Autodesk Fusion 360 part; units mm, degrees
note: some values were not read from the file. Chosen so that the rebuilt part matches the saved one: a direction. Set by a fixed rule: which sketch regions a step uses.
(part 4 of 8)
sketch "Sketch6" plane through (0, 6, 0) normal (0, 1, 0) x (-1, 0, 0)
  arc A0 (-5.2505, -46.5856) -> (-4.5189, -45.8544) centre (-13.5, -37.5997) ccw
  arc A1 (-4.3782, -45.8479) -> (-4.5189, -45.8544) centre (-4.4452, -45.922) ccw
  line L0 (-4.3782, -45.8479) -> (-4.0905, -46.108)
  spline S0 degree 5 poles (-4.0905, -46.108) (-4.0863, -46.1118) (-4.0778, -46.1193) (-4.0648, -46.1302) (-4.047, -46.1441) (-4.024, -46.1606) (-4.0005, -46.1765) (-3.9766, -46.192) (-3.9526, -46.2074) (-3.9285, -46.2225) (-3.9042, -46.2376) (-3.8798, -46.2524) (-3.8552, -46.267) (-3.8303, -46.2814) (-3.8052, -46.2954) (-3.7799, -46.3091) (-3.7544, -46.3225) (-3.7287, -46.3358) (-3.7029, -46.3489) (-3.677, -46.3618) (-3.6509, -46.3746) (-3.6247, -46.3871) (-3.5984, -46.3995) (-3.5719, -46.4117) (-3.5453, -46.4237) (-3.5185, -46.4355) (-3.4916, -46.4471) (-3.4646, -46.4586) (-3.4374, -46.4699) (-3.4102, -46.4811) (-3.3828, -46.492) (-3.3554, -46.5029) (-3.3278, -46.5135) (-3.3001, -46.524) (-3.2723, -46.5344) (-3.2443, -46.5445) (-3.2163, -46.5546) (-3.1882, -46.5645) (-3.16, -46.5742) (-3.1316, -46.5838) (-3.1032, -46.5932) (-3.0747, -46.6025) (-3.0461, -46.6116) (-3.0174, -46.6206) (-2.9886, -46.6295) (-2.9597, -46.6382) (-2.9307, -46.6468) (-2.9017, -46.6552) (-2.8725, -46.6635) (-2.8433, -46.6716) (-2.8139, -46.6796) (-2.7845, -46.6875) (-2.755, -46.6953) (-2.7255, -46.7029) (-2.6958, -46.7103) (-2.6661, -46.7176) (-2.6363, -46.7248) (-2.6064, -46.7319) (-2.5764, -46.7388) (-2.5464, -46.7456) (-2.5163, -46.7523) (-2.4861, -46.7588) (-2.4558, -46.7652) (-2.4255, -46.7715) (-2.395, -46.7776) (-2.3646, -46.7836) (-2.334, -46.7895) (-2.3034, -46.7953) (-2.2727, -46.8009) (-2.242, -46.8064) (-2.2111, -46.8117) (-2.1864, -46.8159) (-2.1679, -46.819) (-2.1555, -46.821) (-2.1493, -46.8221) knots 0 0 0 0 0 0 0.01428571 0.02857143 0.04285714 0.05714286 0.07142857 0.08571429 0.1 0.11428571 0.12857143 0.14285714 0.15714286 0.17142857 0.18571429 0.2 0.21428571 0.22857143 0.24285714 0.25714286 0.27142857 0.28571429 0.3 0.31428571 0.32857143 0.34285714 0.35714286 0.37142857 0.38571429 0.4 0.41428571 0.42857143 0.44285714 0.45714286 0.47142857 0.48571429 0.5 0.51428571 0.52857143 0.54285714 0.55714286 0.57142857 0.58571429 0.6 0.61428571 0.62857143 0.64285714 0.65714286 0.67142857 0.68571429 0.7 0.71428571 0.72857143 0.74285714 0.75714286 0.77142857 0.78571429 0.8 0.81428571 0.82857143 0.84285714 0.85714286 0.87142857 0.88571429 0.9 0.91428571 0.92857143 0.94285714 0.95714286 0.97142857 0.98571429 1 1 1 1 1 1
  arc A2 (-2.1493, -46.8221) -> (-1.6591, -46.1836) centre (-13.5, -37.5997) ccw
  spline S1 degree 5 poles (-1.6591, -46.1836) (-1.6617, -46.1779) (-1.6668, -46.1665) (-1.6746, -46.1493) (-1.685, -46.1265) (-1.6982, -46.0981) (-1.7114, -46.0698) (-1.7248, -46.0416) (-1.7383, -46.0136) (-1.7518, -45.9856) (-1.7655, -45.9577) (-1.7793, -45.9299) (-1.7932, -45.9022) (-1.8072, -45.8746) (-1.8213, -45.8471) (-1.8355, -45.8197) (-1.8498, -45.7925) (-1.8642, -45.7653) (-1.8788, -45.7383) (-1.8934, -45.7113) (-1.9082, -45.6845) (-1.9231, -45.6578) (-1.938, -45.6312) (-1.9531, -45.6047) (-1.9683, -45.5783) (-1.9836, -45.552) (-1.9991, -45.5259) (-2.0146, -45.4999) (-2.0302, -45.474) (-2.046, -45.4482) (-2.0619, -45.4225) (-2.0779, -45.397) (-2.094, -45.3716) (-2.1102, -45.3463) (-2.1265, -45.3211) (-2.143, -45.2961) (-2.1596, -45.2712) (-2.1763, -45.2465) (-2.1931, -45.2219) (-2.21, -45.1974) (-2.227, -45.173) (-2.2442, -45.1488) (-2.2615, -45.1248) (-2.2789, -45.1009) (-2.2965, -45.0771) (-2.3142, -45.0535) (-2.332, -45.0301) (-2.3499, -45.0068) (-2.368, -44.9837) (-2.3861, -44.9607) (-2.4045, -44.9379) (-2.4229, -44.9152) (-2.4415, -44.8928) (-2.4603, -44.8705) (-2.4792, -44.8485) (-2.4983, -44.8266) (-2.5175, -44.8049) (-2.5368, -44.7833) (-2.5562, -44.7619) (-2.5758, -44.7408) (-2.5956, -44.7199) (-2.6156, -44.6992) (-2.6358, -44.6789) (-2.6563, -44.6589) (-2.677, -44.6392) (-2.6978, -44.6196) (-2.7187, -44.6002) (-2.7397, -44.581) (-2.7608, -44.562) (-2.7822, -44.5434) (-2.8041, -44.5254) (-2.8222, -44.5118) (-2.8361, -44.502) (-2.8455, -44.4958) (-2.8502, -44.4927) knots -1 -1 -1 -1 -1 -1 -0.98571429 -0.97142857 -0.95714286 -0.94285714 -0.92857143 -0.91428571 -0.9 -0.88571429 -0.87142857 -0.85714286 -0.84285714 -0.82857143 -0.81428571 -0.8 -0.78571429 -0.77142857 -0.75714286 -0.74285714 -0.72857143 -0.71428571 -0.7 -0.68571429 -0.67142857 -0.65714286 -0.64285714 -0.62857143 -0.61428571 -0.6 -0.58571429 -0.57142857 -0.55714286 -0.54285714 -0.52857143 -0.51428571 -0.5 -0.48571429 -0.47142857 -0.45714286 -0.44285714 -0.42857143 -0.41428571 -0.4 -0.38571429 -0.37142857 -0.35714286 -0.34285714 -0.32857143 -0.31428571 -0.3 -0.28571429 -0.27142857 -0.25714286 -0.24285714 -0.22857143 -0.21428571 -0.2 -0.18571429 -0.17142857 -0.15714286 -0.14285714 -0.12857143 -0.11428571 -0.1 -0.08571429 -0.07142857 -0.05714286 -0.04285714 -0.02857143 -0.01428571 0 0 0 0 0 0
  line L1 (-2.8502, -44.4927) -> (-3.1759, -44.2819)
  arc A3 (-3.2059, -44.1443) -> (-3.1759, -44.2819) centre (-3.1215, -44.198) ccw
  arc A4 (-3.2059, -44.1443) -> (-2.6884, -43.2486) centre (-13.5, -37.5997) ccw
  arc A5 (-2.5542, -43.2059) -> (-2.6884, -43.2486) centre (-2.5998, -43.2949) ccw
  line L2 (-2.5542, -43.2059) -> (-2.209, -43.3827)
  spline S2 degree 5 poles (-2.209, -43.3827) (-2.2039, -43.3853) (-2.1938, -43.3904) (-2.1784, -43.3975) (-2.1576, -43.4063) (-2.1311, -43.4163) (-2.1043, -43.4256) (-2.0773, -43.4344) (-2.0501, -43.443) (-2.0229, -43.4514) (-1.9955, -43.4597) (-1.9681, -43.4677) (-1.9406, -43.4755) (-1.9129, -43.4828) (-1.885, -43.4899) (-1.857, -43.4966) (-1.8289, -43.503) (-1.8006, -43.5091) (-1.7723, -43.5151) (-1.7439, -43.5209) (-1.7154, -43.5264) (-1.6869, -43.5318) (-1.6582, -43.5369) (-1.6295, -43.5419) (-1.6007, -43.5466) (-1.5717, -43.551) (-1.5427, -43.5553) (-1.5137, -43.5594) (-1.4845, -43.5633) (-1.4553, -43.567) (-1.4261, -43.5705) (-1.3967, -43.5739) (-1.3673, -43.577) (-1.3378, -43.58) (-1.3083, -43.5828) (-1.2787, -43.5854) (-1.249, -43.5878) (-1.2193, -43.5901) (-1.1895, -43.5922) (-1.1597, -43.5941) (-1.1298, -43.5959) (-1.0998, -43.5975) (-1.0698, -43.5989) (-1.0398, -43.6002) (-1.0097, -43.6013) (-0.9795, -43.6022) (-0.9493, -43.603) (-0.9191, -43.6036) (-0.8888, -43.604) (-0.8584, -43.6043) (-0.828, -43.6045) (-0.7976, -43.6045) (-0.7671, -43.6043) (-0.7365, -43.604) (-0.706, -43.6036) (-0.6753, -43.6029) (-0.6447, -43.6022) (-0.614, -43.6012) (-0.5833, -43.6002) (-0.5525, -43.599) (-0.5217, -43.5976) (-0.4908, -43.5961) (-0.4599, -43.5945) (-0.429, -43.5927) (-0.398, -43.5907) (-0.367, -43.5886) (-0.336, -43.5864) (-0.3049, -43.584) (-0.2738, -43.5815) (-0.2427, -43.5789) (-0.2115, -43.5761) (-0.1866, -43.5737) (-0.1679, -43.5719) (-0.1554, -43.5707) (-0.1491, -43.57) knots 0 0 0 0 0 0 0.01428571 0.02857143 0.04285714 0.05714286 0.07142857 0.08571429 0.1 0.11428571 0.12857143 0.14285714 0.15714286 0.17142857 0.18571429 0.2 0.21428571 0.22857143 0.24285714 0.25714286 0.27142857 0.28571429 0.3 0.31428571 0.32857143 0.34285714 0.35714286 0.37142857 0.38571429 0.4 0.41428571 0.42857143 0.44285714 0.45714286 0.47142857 0.48571429 0.5 0.51428571 0.52857143 0.54285714 0.55714286 0.57142857 0.58571429 0.6 0.61428571 0.62857143 0.64285714 0.65714286 0.67142857 0.68571429 0.7 0.71428571 0.72857143 0.74285714 0.75714286 0.77142857 0.78571429 0.8 0.81428571 0.82857143 0.84285714 0.85714286 0.87142857 0.88571429 0.9 0.91428571 0.92857143 0.94285714 0.95714286 0.97142857 0.98571429 1 1 1 1 1 1
  arc A6 (-0.1491, -43.57) -> (0.1591, -42.8265) centre (-13.5, -37.5997) ccw
  spline S3 degree 5 poles (0.1591, -42.8265) (0.1551, -42.8216) (0.1472, -42.8119) (0.1353, -42.7974) (0.1193, -42.778) (0.0992, -42.754) (0.0791, -42.7301) (0.0589, -42.7063) (0.0386, -42.6827) (0.0183, -42.6592) (-0.0021, -42.6358) (-0.0227, -42.6125) (-0.0432, -42.5893) (-0.0639, -42.5663) (-0.0846, -42.5434) (-0.1055, -42.5206) (-0.1263, -42.498) (-0.1473, -42.4755) (-0.1684, -42.4531) (-0.1895, -42.4309) (-0.2107, -42.4088) (-0.232, -42.3869) (-0.2533, -42.365) (-0.2747, -42.3433) (-0.2963, -42.3218) (-0.3178, -42.3004) (-0.3395, -42.2791) (-0.3612, -42.258) (-0.3831, -42.2371) (-0.405, -42.2162) (-0.4269, -42.1956) (-0.449, -42.175) (-0.4711, -42.1547) (-0.4933, -42.1344) (-0.5156, -42.1144) (-0.538, -42.0945) (-0.5605, -42.0747) (-0.583, -42.0551) (-0.6056, -42.0357) (-0.6283, -42.0164) (-0.651, -41.9973) (-0.6739, -41.9784) (-0.6968, -41.9597) (-0.7198, -41.9411) (-0.7429, -41.9227) (-0.7661, -41.9045) (-0.7894, -41.8864) (-0.8127, -41.8685) (-0.8362, -41.8509) (-0.8597, -41.8334) (-0.8833, -41.8161) (-0.907, -41.799) (-0.9308, -41.7822) (-0.9547, -41.7655) (-0.9786, -41.7491) (-1.0027, -41.7329) (-1.0268, -41.7169) (-1.0511, -41.701) (-1.0754, -41.6854) (-1.0998, -41.6701) (-1.1243, -41.655) (-1.149, -41.6402) (-1.1738, -41.6258) (-1.1987, -41.6118) (-1.2238, -41.5981) (-1.249, -41.5846) (-1.2742, -41.5713) (-1.2994, -41.5581) (-1.3248, -41.5452) (-1.3503, -41.5328) (-1.3761, -41.5211) (-1.397, -41.5126) (-1.413, -41.5068) (-1.4237, -41.5032) (-1.4291, -41.5015) knots -1 -1 -1 -1 -1 -1 -0.98571429 -0.97142857 -0.95714286 -0.94285714 -0.92857143 -0.91428571 -0.9 -0.88571429 -0.87142857 -0.85714286 -0.84285714 -0.82857143 -0.81428571 -0.8 -0.78571429 -0.77142857 -0.75714286 -0.74285714 -0.72857143 -0.71428571 -0.7 -0.68571429 -0.67142857 -0.65714286 -0.64285714 -0.62857143 -0.61428571 -0.6 -0.58571429 -0.57142857 -0.55714286 -0.54285714 -0.52857143 -0.51428571 -0.5 -0.48571429 -0.47142857 -0.45714286 -0.44285714 -0.42857143 -0.41428571 -0.4 -0.38571429 -0.37142857 -0.35714286 -0.34285714 -0.32857143 -0.31428571 -0.3 -0.28571429 -0.27142857 -0.25714286 -0.24285714 -0.22857143 -0.21428571 -0.2 -0.18571429 -0.17142857 -0.15714286 -0.14285714 -0.12857143 -0.11428571 -0.1 -0.08571429 -0.07142857 -0.05714286 -0.04285714 -0.02857143 -0.01428571 0 0 0 0 0 0
  line L3 (-1.4291, -41.5015) -> (-1.7982, -41.3822)
  arc A7 (-1.8628, -41.257) -> (-1.7982, -41.3822) centre (-1.7674, -41.287) ccw
  arc A8 (-1.8628, -41.257) -> (-1.5948, -40.2579) centre (-13.5, -37.5997) ccw
  arc A9 (-1.4762, -40.1819) -> (-1.5948, -40.2579) centre (-1.4972, -40.2797) ccw
  line L4 (-1.4762, -40.1819) -> (-1.0969, -40.2634)
  spline S4 degree 5 poles (-1.0969, -40.2634) (-1.0914, -40.2645) (-1.0803, -40.2668) (-1.0636, -40.2697) (-1.0412, -40.2728) (-1.0131, -40.2757) (-0.9847, -40.2777) (-0.9563, -40.2792) (-0.9279, -40.2805) (-0.8994, -40.2815) (-0.8709, -40.2824) (-0.8423, -40.2831) (-0.8137, -40.2834) (-0.785, -40.2834) (-0.7563, -40.283) (-0.7275, -40.2822) (-0.6987, -40.2811) (-0.6698, -40.2798) (-0.6409, -40.2782) (-0.612, -40.2764) (-0.583, -40.2744) (-0.5541, -40.2722) (-0.5251, -40.2698) (-0.496, -40.2671) (-0.467, -40.2641) (-0.4379, -40.261) (-0.4088, -40.2576) (-0.3796, -40.254) (-0.3505, -40.2503) (-0.3213, -40.2463) (-0.2921, -40.2421) (-0.2629, -40.2377) (-0.2337, -40.2332) (-0.2044, -40.2284) (-0.1752, -40.2235) (-0.1459, -40.2183) (-0.1166, -40.213) (-0.0873, -40.2075) (-0.058, -40.2018) (-0.0287, -40.196) (0.0006, -40.1899) (0.03, -40.1837) (0.0593, -40.1773) (0.0887, -40.1708) (0.118, -40.164) (0.1474, -40.1571) (0.1768, -40.1501) (0.2062, -40.1428) (0.2356, -40.1354) (0.265, -40.1279) (0.2944, -40.1201) (0.3238, -40.1122) (0.3532, -40.1042) (0.3826, -40.096) (0.412, -40.0876) (0.4414, -40.0791) (0.4708, -40.0704) (0.5002, -40.0616) (0.5297, -40.0526) (0.5591, -40.0435) (0.5885, -40.0342) (0.6179, -40.0248) (0.6473, -40.0152) (0.6767, -40.0054) (0.7061, -39.9955) (0.7355, -39.9855) (0.7649, -39.9753) (0.7943, -39.965) (0.8237, -39.9545) (0.8531, -39.9439) (0.8825, -39.9331) (0.906, -39.9244) (0.9236, -39.9178) (0.9353, -39.9134) (0.9412, -39.9111) knots 0 0 0 0 0 0 0.01428571 0.02857143 0.04285714 0.05714286 0.07142857 0.08571429 0.1 0.11428571 0.12857143 0.14285714 0.15714286 0.17142857 0.18571429 0.2 0.21428571 0.22857143 0.24285714 0.25714286 0.27142857 0.28571429 0.3 0.31428571 0.32857143 0.34285714 0.35714286 0.37142857 0.38571429 0.4 0.41428571 0.42857143 0.44285714 0.45714286 0.47142857 0.48571429 0.5 0.51428571 0.52857143 0.54285714 0.55714286 0.57142857 0.58571429 0.6 0.61428571 0.62857143 0.64285714 0.65714286 0.67142857 0.68571429 0.7 0.71428571 0.72857143 0.74285714 0.75714286 0.77142857 0.78571429 0.8 0.81428571 0.82857143 0.84285714 0.85714286 0.87142857 0.88571429 0.9 0.91428571 0.92857143 0.94285714 0.95714286 0.97142857 0.98571429 1 1 1 1 1 1
  arc A10 (0.9412, -39.9111) -> (1.0465, -39.1132) centre (-13.5, -37.5997) ccw
  spline S5 degree 5 poles (1.0465, -39.1132) (1.0414, -39.1095) (1.0312, -39.1021) (1.0159, -39.0912) (0.9955, -39.0767) (0.9699, -39.0587) (0.9443, -39.0408) (0.9186, -39.023) (0.8929, -39.0054) (0.8671, -38.988) (0.8413, -38.9707) (0.8155, -38.9535) (0.7896, -38.9364) (0.7637, -38.9196) (0.7378, -38.9028) (0.7118, -38.8862) (0.6857, -38.8698) (0.6597, -38.8534) (0.6335, -38.8373) (0.6074, -38.8213) (0.5812, -38.8054) (0.5549, -38.7897) (0.5287, -38.7742) (0.5024, -38.7588) (0.476, -38.7435) (0.4496, -38.7284) (0.4232, -38.7135) (0.3967, -38.6987) (0.3702, -38.6841) (0.3437, -38.6697) (0.3171, -38.6554) (0.2905, -38.6413) (0.2638, -38.6273) (0.2371, -38.6135) (0.2104, -38.5999) (0.1837, -38.5865) (0.1569, -38.5732) (0.13, -38.5601) (0.1032, -38.5472) (0.0763, -38.5345) (0.0493, -38.5219) (0.0224, -38.5096) (-0.0047, -38.4974) (-0.0317, -38.4854) (-0.0588, -38.4736) (-0.0859, -38.462) (-0.113, -38.4506) (-0.1402, -38.4394) (-0.1674, -38.4284) (-0.1946, -38.4176) (-0.2219, -38.407) (-0.2492, -38.3966) (-0.2766, -38.3865) (-0.3039, -38.3766) (-0.3313, -38.3669) (-0.3588, -38.3575) (-0.3863, -38.3483) (-0.4138, -38.3393) (-0.4413, -38.3305) (-0.4688, -38.322) (-0.4964, -38.3137) (-0.5241, -38.3059) (-0.5518, -38.2984) (-0.5795, -38.2913) (-0.6073, -38.2845) (-0.635, -38.278) (-0.6628, -38.2717) (-0.6906, -38.2655) (-0.7185, -38.2596) (-0.7463, -38.2542) (-0.7743, -38.2496) (-0.7967, -38.2468) (-0.8136, -38.2453) (-0.8249, -38.2446) (-0.8305, -38.2443) knots -1 -1 -1 -1 -1 -1 -0.98571429 -0.97142857 -0.95714286 -0.94285714 -0.92857143 -0.91428571 -0.9 -0.88571429 -0.87142857 -0.85714286 -0.84285714 -0.82857143 -0.81428571 -0.8 -0.78571429 -0.77142857 -0.75714286 -0.74285714 -0.72857143 -0.71428571 -0.7 -0.68571429 -0.67142857 -0.65714286 -0.64285714 -0.62857143 -0.61428571 -0.6 -0.58571429 -0.57142857 -0.55714286 -0.54285714 -0.52857143 -0.51428571 -0.5 -0.48571429 -0.47142857 -0.45714286 -0.44285714 -0.42857143 -0.41428571 -0.4 -0.38571429 -0.37142857 -0.35714286 -0.34285714 -0.32857143 -0.31428571 -0.3 -0.28571429 -0.27142857 -0.25714286 -0.24285714 -0.22857143 -0.21428571 -0.2 -0.18571429 -0.17142857 -0.15714286 -0.14285714 -0.12857143 -0.11428571 -0.1 -0.08571429 -0.07142857 -0.05714286 -0.04285714 -0.02857143 -0.01428571 0 0 0 0 0 0
  line L5 (-0.8305, -38.2443) -> (-1.2179, -38.2246)
  arc A11 (-1.3127, -38.1205) -> (-1.2179, -38.2246) centre (-1.2128, -38.1247) ccw
  arc A12 (-1.3127, -38.1205) -> (-1.3124, -37.086) centre (-13.5, -37.5997) ccw
  arc A13 (-1.2176, -36.9819) -> (-1.3124, -37.086) centre (-1.2125, -37.0818) ccw
  line L6 (-1.2176, -36.9819) -> (-0.8302, -36.9624)
  spline S6 degree 5 poles (-0.8302, -36.9624) (-0.8245, -36.9622) (-0.8132, -36.9615) (-0.7963, -36.96) (-0.7739, -36.9572) (-0.746, -36.9526) (-0.7181, -36.9472) (-0.6903, -36.9414) (-0.6625, -36.9352) (-0.6347, -36.9289) (-0.6069, -36.9224) (-0.5791, -36.9156) (-0.5514, -36.9085) (-0.5237, -36.9011) (-0.496, -36.8932) (-0.4684, -36.885) (-0.4409, -36.8765) (-0.4133, -36.8677) (-0.3858, -36.8587) (-0.3584, -36.8495) (-0.3309, -36.8401) (-0.3035, -36.8305) (-0.2761, -36.8206) (-0.2488, -36.8105) (-0.2214, -36.8002) (-0.1942, -36.7896) (-0.1669, -36.7788) (-0.1397, -36.7678) (-0.1125, -36.7566) (-0.0854, -36.7452) (-0.0583, -36.7336) (-0.0312, -36.7218) (-0.0041, -36.7099) (0.0229, -36.6977) (0.0499, -36.6854) (0.0768, -36.6728) (0.1037, -36.6601) (0.1306, -36.6472) (0.1574, -36.6341) (0.1842, -36.6209) (0.211, -36.6074) (0.2377, -36.5938) (0.2644, -36.5801) (0.2911, -36.5661) (0.3177, -36.552) (0.3443, -36.5378) (0.3708, -36.5233) (0.3974, -36.5087) (0.4238, -36.494) (0.4503, -36.4791) (0.4767, -36.464) (0.503, -36.4488) (0.5293, -36.4334) (0.5556, -36.4179) (0.5819, -36.4022) (0.6081, -36.3863) (0.6343, -36.3703) (0.6604, -36.3542) (0.6865, -36.3379) (0.7125, -36.3215) (0.7385, -36.3049) (0.7645, -36.2881) (0.7904, -36.2713) (0.8163, -36.2542) (0.8421, -36.2371) (0.8679, -36.2198) (0.8937, -36.2023) (0.9194, -36.1847) (0.9451, -36.167) (0.9707, -36.1492) (0.9963, -36.1312) (1.0168, -36.1166) (1.0321, -36.1057) (1.0423, -36.0984) (1.0474, -36.0947) knots 0 0 0 0 0 0 0.01428571 0.02857143 0.04285714 0.05714286 0.07142857 0.08571429 0.1 0.11428571 0.12857143 0.14285714 0.15714286 0.17142857 0.18571429 0.2 0.21428571 0.22857143 0.24285714 0.25714286 0.27142857 0.28571429 0.3 0.31428571 0.32857143 0.34285714 0.35714286 0.37142857 0.38571429 0.4 0.41428571 0.42857143 0.44285714 0.45714286 0.47142857 0.48571429 0.5 0.51428571 0.52857143 0.54285714 0.55714286 0.57142857 0.58571429 0.6 0.61428571 0.62857143 0.64285714 0.65714286 0.67142857 0.68571429 0.7 0.71428571 0.72857143 0.74285714 0.75714286 0.77142857 0.78571429 0.8 0.81428571 0.82857143 0.84285714 0.85714286 0.87142857 0.88571429 0.9 0.91428571 0.92857143 0.94285714 0.95714286 0.97142857 0.98571429 1 1 1 1 1 1
  arc A14 (1.0474, -36.0947) -> (0.9425, -35.2967) centre (-13.5, -37.5997) ccw
  spline S7 degree 5 poles (0.9425, -35.2967) (0.9367, -35.2944) (0.9249, -35.29) (0.9073, -35.2834) (0.8838, -35.2746) (0.8544, -35.2639) (0.8251, -35.2532) (0.7957, -35.2427) (0.7663, -35.2324) (0.7369, -35.2222) (0.7075, -35.2121) (0.6781, -35.2022) (0.6487, -35.1925) (0.6193, -35.1829) (0.5899, -35.1734) (0.5605, -35.1641) (0.5311, -35.1549) (0.5017, -35.1459) (0.4723, -35.1371) (0.4428, -35.1284) (0.4134, -35.1199) (0.384, -35.1115) (0.3546, -35.1033) (0.3252, -35.0952) (0.2958, -35.0873) (0.2664, -35.0795) (0.237, -35.072) (0.2076, -35.0646) (0.1783, -35.0573) (0.1489, -35.0502) (0.1195, -35.0433) (0.0902, -35.0366) (0.0608, -35.03) (0.0315, -35.0236) (0.0021, -35.0173) (-0.0272, -35.0113) (-0.0565, -35.0054) (-0.0858, -34.9997) (-0.1151, -34.9942) (-0.1444, -34.9888) (-0.1737, -34.9837) (-0.2029, -34.9787) (-0.2322, -34.9739) (-0.2614, -34.9694) (-0.2906, -34.965) (-0.3198, -34.9608) (-0.3489, -34.9568) (-0.3781, -34.953) (-0.4072, -34.9494) (-0.4363, -34.946) (-0.4654, -34.9428) (-0.4945, -34.9399) (-0.5235, -34.9372) (-0.5525, -34.9347) (-0.5815, -34.9325) (-0.6104, -34.9305) (-0.6394, -34.9287) (-0.6682, -34.9271) (-0.6971, -34.9257) (-0.7259, -34.9246) (-0.7547, -34.9238) (-0.7835, -34.9234) (-0.8121, -34.9233) (-0.8408, -34.9237) (-0.8693, -34.9243) (-0.8979, -34.9252) (-0.9263, -34.9263) (-0.9548, -34.9275) (-0.9832, -34.929) (-1.0115, -34.931) (-1.0397, -34.9338) (-1.0621, -34.9369) (-1.0788, -34.9398) (-1.0899, -34.9421) (-1.0954, -34.9433) knots -1 -1 -1 -1 -1 -1 -0.98571429 -0.97142857 -0.95714286 -0.94285714 -0.92857143 -0.91428571 -0.9 -0.88571429 -0.87142857 -0.85714286 -0.84285714 -0.82857143 -0.81428571 -0.8 -0.78571429 -0.77142857 -0.75714286 -0.74285714 -0.72857143 -0.71428571 -0.7 -0.68571429 -0.67142857 -0.65714286 -0.64285714 -0.62857143 -0.61428571 -0.6 -0.58571429 -0.57142857 -0.55714286 -0.54285714 -0.52857143 -0.51428571 -0.5 -0.48571429 -0.47142857 -0.45714286 -0.44285714 -0.42857143 -0.41428571 -0.4 -0.38571429 -0.37142857 -0.35714286 -0.34285714 -0.32857143 -0.31428571 -0.3 -0.28571429 -0.27142857 -0.25714286 -0.24285714 -0.22857143 -0.21428571 -0.2 -0.18571429 -0.17142857 -0.15714286 -0.14285714 -0.12857143 -0.11428571 -0.1 -0.08571429 -0.07142857 -0.05714286 -0.04285714 -0.02857143 -0.01428571 0 0 0 0 0 0
  line L7 (-1.0954, -34.9433) -> (-1.4747, -35.0245)
  arc A15 (-1.5932, -34.9484) -> (-1.4747, -35.0245) centre (-1.4956, -34.9267) ccw
  arc A16 (-1.5932, -34.9484) -> (-1.8607, -33.9492) centre (-13.5, -37.5997) ccw
  arc A17 (-1.796, -33.8241) -> (-1.8607, -33.9492) centre (-1.7653, -33.9192) ccw
  line L8 (-1.796, -33.8241) -> (-1.4268, -33.705)
  spline S8 degree 5 poles (-1.4268, -33.705) (-1.4214, -33.7032) (-1.4107, -33.6996) (-1.3948, -33.6938) (-1.3738, -33.6853) (-1.348, -33.6737) (-1.3225, -33.6613) (-1.2971, -33.6484) (-1.2719, -33.6353) (-1.2466, -33.6219) (-1.2215, -33.6085) (-1.1964, -33.5948) (-1.1715, -33.5807) (-1.1467, -33.5664) (-1.122, -33.5516) (-1.0974, -33.5366) (-1.073, -33.5212) (-1.0487, -33.5056) (-1.0245, -33.4898) (-1.0003, -33.4738) (-0.9762, -33.4576) (-0.9522, -33.4412) (-0.9283, -33.4246) (-0.9045, -33.4077) (-0.8808, -33.3907) (-0.8572, -33.3734) (-0.8337, -33.3559) (-0.8103, -33.3382) (-0.7869, -33.3204) (-0.7636, -33.3024) (-0.7404, -33.2841) (-0.7173, -33.2658) (-0.6943, -33.2472) (-0.6714, -33.2285) (-0.6485, -33.2095) (-0.6257, -33.1905) (-0.603, -33.1712) (-0.5804, -33.1518) (-0.5579, -33.1322) (-0.5354, -33.1125) (-0.513, -33.0926) (-0.4907, -33.0725) (-0.4685, -33.0523) (-0.4463, -33.032) (-0.4243, -33.0115) (-0.4023, -32.9908) (-0.3804, -32.97) (-0.3586, -32.949) (-0.3368, -32.9279) (-0.3151, -32.9067) (-0.2935, -32.8853) (-0.272, -32.8637) (-0.2506, -32.8421) (-0.2292, -32.8203) (-0.2079, -32.7983) (-0.1867, -32.7762) (-0.1655, -32.754) (-0.1445, -32.7317) (-0.1235, -32.7092) (-0.1026, -32.6865) (-0.0818, -32.6638) (-0.061, -32.6409) (-0.0403, -32.6179) (-0.0198, -32.5948) (0.0008, -32.5715) (0.0212, -32.5481) (0.0416, -32.5246) (0.0619, -32.5009) (0.0821, -32.4772) (0.1022, -32.4533) (0.1223, -32.4293) (0.1383, -32.41) (0.1502, -32.3954) (0.1582, -32.3857) (0.1621, -32.3809) knots 0 0 0 0 0 0 0.01428571 0.02857143 0.04285714 0.05714286 0.07142857 0.08571429 0.1 0.11428571 0.12857143 0.14285714 0.15714286 0.17142857 0.18571429 0.2 0.21428571 0.22857143 0.24285714 0.25714286 0.27142857 0.28571429 0.3 0.31428571 0.32857143 0.34285714 0.35714286 0.37142857 0.38571429 0.4 0.41428571 0.42857143 0.44285714 0.45714286 0.47142857 0.48571429 0.5 0.51428571 0.52857143 0.54285714 0.55714286 0.57142857 0.58571429 0.6 0.61428571 0.62857143 0.64285714 0.65714286 0.67142857 0.68571429 0.7 0.71428571 0.72857143 0.74285714 0.75714286 0.77142857 0.78571429 0.8 0.81428571 0.82857143 0.84285714 0.85714286 0.87142857 0.88571429 0.9 0.91428571 0.92857143 0.94285714 0.95714286 0.97142857 0.98571429 1 1 1 1 1 1
  arc A18 (0.1621, -32.3809) -> (-0.1457, -31.6371) centre (-13.5, -37.5997) ccw
  spline S9 degree 5 poles (-0.1457, -31.6371) (-0.1519, -31.6365) (-0.1644, -31.6353) (-0.1831, -31.6334) (-0.2081, -31.6311) (-0.2392, -31.6283) (-0.2704, -31.6256) (-0.3015, -31.6231) (-0.3325, -31.6207) (-0.3636, -31.6184) (-0.3946, -31.6163) (-0.4255, -31.6144) (-0.4564, -31.6125) (-0.4873, -31.6109) (-0.5182, -31.6093) (-0.549, -31.608) (-0.5798, -31.6067) (-0.6105, -31.6057) (-0.6412, -31.6047) (-0.6719, -31.6039) (-0.7025, -31.6033) (-0.7331, -31.6028) (-0.7636, -31.6025) (-0.7941, -31.6023) (-0.8245, -31.6023) (-0.8549, -31.6024) (-0.8853, -31.6027) (-0.9156, -31.6031) (-0.9458, -31.6037) (-0.976, -31.6045) (-1.0062, -31.6054) (-1.0363, -31.6065) (-1.0664, -31.6077) (-1.0964, -31.6091) (-1.1263, -31.6107) (-1.1562, -31.6125) (-1.1861, -31.6144) (-1.2158, -31.6164) (-1.2456, -31.6187) (-1.2752, -31.6211) (-1.3048, -31.6237) (-1.3344, -31.6265) (-1.3639, -31.6294) (-1.3933, -31.6326) (-1.4226, -31.6359) (-1.4519, -31.6394) (-1.4811, -31.6431) (-1.5102, -31.647) (-1.5393, -31.651) (-1.5683, -31.6553) (-1.5972, -31.6598) (-1.626, -31.6645) (-1.6548, -31.6694) (-1.6834, -31.6745) (-1.712, -31.6798) (-1.7405, -31.6854) (-1.7689, -31.6911) (-1.7972, -31.6971) (-1.8254, -31.7032) (-1.8536, -31.7096) (-1.8816, -31.7163) (-1.9094, -31.7233) (-1.9372, -31.7307) (-1.9647, -31.7384) (-1.9922, -31.7464) (-2.0195, -31.7546) (-2.0467, -31.7631) (-2.0739, -31.7716) (-2.1009, -31.7804) (-2.1278, -31.7897) (-2.1542, -31.7997) (-2.1751, -31.8085) (-2.1904, -31.8156) (-2.2006, -31.8207) (-2.2056, -31.8232) knots -1 -1 -1 -1 -1 -1 -0.98571429 -0.97142857 -0.95714286 -0.94285714 -0.92857143 -0.91428571 -0.9 -0.88571429 -0.87142857 -0.85714286 -0.84285714 -0.82857143 -0.81428571 -0.8 -0.78571429 -0.77142857 -0.75714286 -0.74285714 -0.72857143 -0.71428571 -0.7 -0.68571429 -0.67142857 -0.65714286 -0.64285714 -0.62857143 -0.61428571 -0.6 -0.58571429 -0.57142857 -0.55714286 -0.54285714 -0.52857143 -0.51428571 -0.5 -0.48571429 -0.47142857 -0.45714286 -0.44285714 -0.42857143 -0.41428571 -0.4 -0.38571429 -0.37142857 -0.35714286 -0.34285714 -0.32857143 -0.31428571 -0.3 -0.28571429 -0.27142857 -0.25714286 -0.24285714 -0.22857143 -0.21428571 -0.2 -0.18571429 -0.17142857 -0.15714286 -0.14285714 -0.12857143 -0.11428571 -0.1 -0.08571429 -0.07142857 -0.05714286 -0.04285714 -0.02857143 -0.01428571 0 0 0 0 0 0
  line L9 (-2.2056, -31.8232) -> (-2.551, -31.9999)
  arc A19 (-2.6851, -31.9571) -> (-2.551, -31.9999) centre (-2.5965, -31.9108) ccw
  arc A20 (-2.6851, -31.9571) -> (-3.2021, -31.0611) centre (-13.5, -37.5997) ccw
  arc A21 (-3.172, -30.9235) -> (-3.2021, -31.0611) centre (-3.1177, -31.0075) ccw
  line L10 (-3.172, -30.9235) -> (-2.8462, -30.7129)
  spline S10 degree 5 poles (-2.8462, -30.7129) (-2.8415, -30.7098) (-2.8321, -30.7036) (-2.8182, -30.6938) (-2.8001, -30.6802) (-2.7782, -30.6623) (-2.7568, -30.6437) (-2.7356, -30.6247) (-2.7146, -30.6055) (-2.6937, -30.5861) (-2.6729, -30.5666) (-2.6522, -30.5468) (-2.6317, -30.5268) (-2.6115, -30.5065) (-2.5915, -30.4859) (-2.5717, -30.465) (-2.5521, -30.4438) (-2.5326, -30.4225) (-2.5133, -30.4009) (-2.4941, -30.3792) (-2.475, -30.3573) (-2.4561, -30.3353) (-2.4373, -30.313) (-2.4187, -30.2906) (-2.4002, -30.268) (-2.3819, -30.2452) (-2.3637, -30.2222) (-2.3456, -30.1991) (-2.3277, -30.1758) (-2.3099, -30.1524) (-2.2922, -30.1288) (-2.2746, -30.105) (-2.2572, -30.0812) (-2.2398, -30.0571) (-2.2227, -30.0329) (-2.2056, -30.0086) (-2.1887, -29.9841) (-2.1718, -29.9595) (-2.1551, -29.9348) (-2.1385, -29.9099) (-2.1221, -29.8849) (-2.1057, -29.8597) (-2.0895, -29.8345) (-2.0734, -29.8091) (-2.0574, -29.7836) (-2.0415, -29.7579) (-2.0257, -29.7321) (-2.01, -29.7062) (-1.9945, -29.6802) (-1.979, -29.6541) (-1.9637, -29.6278) (-1.9485, -29.6015) (-1.9334, -29.575) (-1.9184, -29.5484) (-1.9035, -29.5217) (-1.8887, -29.4948) (-1.8741, -29.4679) (-1.8595, -29.4409) (-1.8451, -29.4137) (-1.8307, -29.3865) (-1.8165, -29.3591) (-1.8024, -29.3316) (-1.7884, -29.304) (-1.7745, -29.2764) (-1.7607, -29.2486) (-1.747, -29.2207) (-1.7334, -29.1927) (-1.7199, -29.1646) (-1.7065, -29.1364) (-1.6933, -29.1081) (-1.6801, -29.0798) (-1.6697, -29.057) (-1.6619, -29.0398) (-1.6567, -29.0284) (-1.6541, -29.0227) knots 0 0 0 0 0 0 0.01428571 0.02857143 0.04285714 0.05714286 0.07142857 0.08571429 0.1 0.11428571 0.12857143 0.14285714 0.15714286 0.17142857 0.18571429 0.2 0.21428571 0.22857143 0.24285714 0.25714286 0.27142857 0.28571429 0.3 0.31428571 0.32857143 0.34285714 0.35714286 0.37142857 0.38571429 0.4 0.41428571 0.42857143 0.44285714 0.45714286 0.47142857 0.48571429 0.5 0.51428571 0.52857143 0.54285714 0.55714286 0.57142857 0.58571429 0.6 0.61428571 0.62857143 0.64285714 0.65714286 0.67142857 0.68571429 0.7 0.71428571 0.72857143 0.74285714 0.75714286 0.77142857 0.78571429 0.8 0.81428571 0.82857143 0.84285714 0.85714286 0.87142857 0.88571429 0.9 0.91428571 0.92857143 0.94285714 0.95714286 0.97142857 0.98571429 1 1 1 1 1 1
  arc A22 (-1.6541, -29.0227) -> (-2.1439, -28.384) centre (-13.5, -37.5997) ccw
  spline S11 degree 5 poles (-2.1439, -28.384) (-2.1501, -28.385) (-2.1625, -28.387) (-2.1811, -28.3901) (-2.2058, -28.3942) (-2.2366, -28.3996) (-2.2674, -28.4051) (-2.2981, -28.4107) (-2.3287, -28.4164) (-2.3592, -28.4223) (-2.3897, -28.4283) (-2.4201, -28.4344) (-2.4505, -28.4406) (-2.4808, -28.447) (-2.511, -28.4535) (-2.5411, -28.4602) (-2.5711, -28.4669) (-2.6011, -28.4738) (-2.631, -28.4809) (-2.6608, -28.4881) (-2.6905, -28.4954) (-2.7202, -28.5028) (-2.7498, -28.5104) (-2.7793, -28.5181) (-2.8087, -28.526) (-2.838, -28.534) (-2.8673, -28.5421) (-2.8964, -28.5504) (-2.9255, -28.5588) (-2.9545, -28.5673) (-2.9834, -28.576) (-3.0122, -28.5849) (-3.0409, -28.5939) (-3.0695, -28.603) (-3.098, -28.6123) (-3.1264, -28.6217) (-3.1548, -28.6312) (-3.183, -28.6409) (-3.2111, -28.6508) (-3.2392, -28.6608) (-3.2671, -28.671) (-3.2949, -28.6813) (-3.3226, -28.6918) (-3.3502, -28.7025) (-3.3777, -28.7133) (-3.405, -28.7242) (-3.4323, -28.7354) (-3.4595, -28.7466) (-3.4865, -28.7581) (-3.5134, -28.7697) (-3.5402, -28.7815) (-3.5668, -28.7935) (-3.5933, -28.8057) (-3.6196, -28.818) (-3.6458, -28.8306) (-3.6719, -28.8433) (-3.6979, -28.8562) (-3.7237, -28.8693) (-3.7494, -28.8825) (-3.7749, -28.896) (-3.8002, -28.9097) (-3.8253, -28.9237) (-3.8502, -28.938) (-3.8748, -28.9526) (-3.8992, -28.9674) (-3.9235, -28.9824) (-3.9476, -28.9976) (-3.9716, -29.0129) (-3.9955, -29.0284) (-4.019, -29.0443) (-4.042, -29.0608) (-4.0598, -29.0747) (-4.0728, -29.0856) (-4.0813, -29.0931) (-4.0855, -29.0969) knots -1 -1 -1 -1 -1 -1 -0.98571429 -0.97142857 -0.95714286 -0.94285714 -0.92857143 -0.91428571 -0.9 -0.88571429 -0.87142857 -0.85714286 -0.84285714 -0.82857143 -0.81428571 -0.8 -0.78571429 -0.77142857 -0.75714286 -0.74285714 -0.72857143 -0.71428571 -0.7 -0.68571429 -0.67142857 -0.65714286 -0.64285714 -0.62857143 -0.61428571 -0.6 -0.58571429 -0.57142857 -0.55714286 -0.54285714 -0.52857143 -0.51428571 -0.5 -0.48571429 -0.47142857 -0.45714286 -0.44285714 -0.42857143 -0.41428571 -0.4 -0.38571429 -0.37142857 -0.35714286 -0.34285714 -0.32857143 -0.31428571 -0.3 -0.28571429 -0.27142857 -0.25714286 -0.24285714 -0.22857143 -0.21428571 -0.2 -0.18571429 -0.17142857 -0.15714286 -0.14285714 -0.12857143 -0.11428571 -0.1 -0.08571429 -0.07142857 -0.05714286 -0.04285714 -0.02857143 -0.01428571 0 0 0 0 0 0
  line L11 (-4.0855, -29.0969) -> (-4.3734, -29.3568)
  arc A23 (-4.5141, -29.3503) -> (-4.3734, -29.3568) centre (-4.4404, -29.2826) ccw
  arc A24 (-4.5141, -29.3503) -> (-5.2453, -28.6186) centre (-13.5, -37.5997) ccw
  arc A25 (-5.2518, -28.4779) -> (-5.2453, -28.6186) centre (-5.1777, -28.5449) ccw
  line L12 (-5.2518, -28.4779) -> (-4.9917, -28.1902)
  spline S12 degree 5 poles (-4.9917, -28.1902) (-4.9879, -28.186) (-4.9804, -28.1775) (-4.9695, -28.1645) (-4.9556, -28.1467) (-4.9391, -28.1237) (-4.9232, -28.1002) (-4.9077, -28.0763) (-4.8924, -28.0523) (-4.8772, -28.0282) (-4.8621, -28.0039) (-4.8473, -27.9795) (-4.8327, -27.9549) (-4.8184, -27.9301) (-4.8044, -27.905) (-4.7906, -27.8796) (-4.7772, -27.8541) (-4.7639, -27.8285) (-4.7508, -27.8026) (-4.7379, -27.7767) (-4.7252, -27.7506) (-4.7126, -27.7244) (-4.7002, -27.6981) (-4.688, -27.6716) (-4.676, -27.645) (-4.6642, -27.6182) (-4.6526, -27.5913) (-4.6411, -27.5643) (-4.6298, -27.5372) (-4.6187, -27.5099) (-4.6077, -27.4825) (-4.5969, -27.4551) (-4.5862, -27.4275) (-4.5757, -27.3998) (-4.5654, -27.372) (-4.5552, -27.3441) (-4.5451, -27.316) (-4.5353, -27.2879) (-4.5255, -27.2597) (-4.5159, -27.2314) (-4.5065, -27.2029) (-4.4972, -27.1744) (-4.4881, -27.1458) (-4.4791, -27.1171) (-4.4702, -27.0883) (-4.4615, -27.0594) (-4.4529, -27.0304) (-4.4445, -27.0014) (-4.4362, -26.9722) (-4.4281, -26.943) (-4.4201, -26.9137) (-4.4122, -26.8842) (-4.4045, -26.8548) (-4.3969, -26.8252) (-4.3894, -26.7955) (-4.3821, -26.7658) (-4.3749, -26.736) (-4.3678, -26.7061) (-4.3609, -26.6761) (-4.3541, -26.6461) (-4.3474, -26.616) (-4.3409, -26.5858) (-4.3345, -26.5555) (-4.3282, -26.5252) (-4.3221, -26.4948) (-4.3161, -26.4643) (-4.3102, -26.4337) (-4.3045, -26.4031) (-4.2988, -26.3724) (-4.2933, -26.3417) (-4.288, -26.3108) (-4.2838, -26.2861) (-4.2807, -26.2676) (-4.2787, -26.2552) (-4.2777, -26.249) knots 0 0 0 0 0 0 0.01428571 0.02857143 0.04285714 0.05714286 0.07142857 0.08571429 0.1 0.11428571 0.12857143 0.14285714 0.15714286 0.17142857 0.18571429 0.2 0.21428571 0.22857143 0.24285714 0.25714286 0.27142857 0.28571429 0.3 0.31428571 0.32857143 0.34285714 0.35714286 0.37142857 0.38571429 0.4 0.41428571 0.42857143 0.44285714 0.45714286 0.47142857 0.48571429 0.5 0.51428571 0.52857143 0.54285714 0.55714286 0.57142857 0.58571429 0.6 0.61428571 0.62857143 0.64285714 0.65714286 0.67142857 0.68571429 0.7 0.71428571 0.72857143 0.74285714 0.75714286 0.77142857 0.78571429 0.8 0.81428571 0.82857143 0.84285714 0.85714286 0.87142857 0.88571429 0.9 0.91428571 0.92857143 0.94285714 0.95714286 0.97142857 0.98571429 1 1 1 1 1 1
  arc A26 (-4.2777, -26.249) -> (-4.9161, -25.7588) centre (-13.5, -37.5997) ccw
  spline S13 degree 5 poles (-4.9161, -25.7588) (-4.9218, -25.7614) (-4.9333, -25.7665) (-4.9504, -25.7743) (-4.9732, -25.7848) (-5.0016, -25.7979) (-5.0299, -25.8111) (-5.0581, -25.8245) (-5.0862, -25.838) (-5.1142, -25.8515) (-5.1421, -25.8652) (-5.1698, -25.879) (-5.1975, -25.8929) (-5.2251, -25.9069) (-5.2526, -25.921) (-5.28, -25.9352) (-5.3072, -25.9495) (-5.3344, -25.964) (-5.3615, -25.9785) (-5.3884, -25.9931) (-5.4152, -26.0079) (-5.442, -26.0228) (-5.4686, -26.0378) (-5.4951, -26.0528) (-5.5214, -26.068) (-5.5477, -26.0834) (-5.5738, -26.0988) (-5.5999, -26.1143) (-5.6258, -26.13) (-5.6515, -26.1457) (-5.6772, -26.1616) (-5.7027, -26.1776) (-5.7281, -26.1937) (-5.7534, -26.2099) (-5.7786, -26.2263) (-5.8036, -26.2427) (-5.8285, -26.2593) (-5.8532, -26.276) (-5.8779, -26.2928) (-5.9023, -26.3097) (-5.9267, -26.3268) (-5.9509, -26.3439) (-5.9749, -26.3612) (-5.9988, -26.3787) (-6.0226, -26.3962) (-6.0462, -26.4139) (-6.0696, -26.4317) (-6.0929, -26.4496) (-6.1161, -26.4677) (-6.139, -26.4859) (-6.1619, -26.5042) (-6.1845, -26.5226) (-6.2069, -26.5413) (-6.2292, -26.56) (-6.2512, -26.5789) (-6.2731, -26.598) (-6.2948, -26.6172) (-6.3164, -26.6365) (-6.3378, -26.6559) (-6.3589, -26.6755) (-6.3799, -26.6953) (-6.4005, -26.7153) (-6.4208, -26.7356) (-6.4408, -26.756) (-6.4606, -26.7767) (-6.4801, -26.7975) (-6.4995, -26.8184) (-6.5187, -26.8394) (-6.5378, -26.8605) (-6.5564, -26.882) (-6.5743, -26.9039) (-6.5879, -26.9219) (-6.5977, -26.9358) (-6.6039, -26.9452) (-6.607, -26.9499) knots -1 -1 -1 -1 -1 -1 -0.98571429 -0.97142857 -0.95714286 -0.94285714 -0.92857143 -0.91428571 -0.9 -0.88571429 -0.87142857 -0.85714286 -0.84285714 -0.82857143 -0.81428571 -0.8 -0.78571429 -0.77142857 -0.75714286 -0.74285714 -0.72857143 -0.71428571 -0.7 -0.68571429 -0.67142857 -0.65714286 -0.64285714 -0.62857143 -0.61428571 -0.6 -0.58571429 -0.57142857 -0.55714286 -0.54285714 -0.52857143 -0.51428571 -0.5 -0.48571429 -0.47142857 -0.45714286 -0.44285714 -0.42857143 -0.41428571 -0.4 -0.38571429 -0.37142857 -0.35714286 -0.34285714 -0.32857143 -0.31428571 -0.3 -0.28571429 -0.27142857 -0.25714286 -0.24285714 -0.22857143 -0.21428571 -0.2 -0.18571429 -0.17142857 -0.15714286 -0.14285714 -0.12857143 -0.11428571 -0.1 -0.08571429 -0.07142857 -0.05714286 -0.04285714 -0.02857143 -0.01428571 0 0 0 0 0 0
  line L13 (-6.607, -26.9499) -> (-6.8178, -27.2756)
  arc A27 (-6.9554, -27.3056) -> (-6.8178, -27.2756) centre (-6.9017, -27.2212) ccw
  arc A28 (-6.9554, -27.3056) -> (-7.8511, -26.7881) centre (-13.5, -37.5997) ccw
  arc A29 (-7.8938, -26.6539) -> (-7.8511, -26.7881) centre (-7.8048, -26.6995) ccw
  line L14 (-7.8938, -26.6539) -> (-7.717, -26.3087)
  spline S14 degree 5 poles (-7.717, -26.3087) (-7.7144, -26.3036) (-7.7094, -26.2935) (-7.7022, -26.2781) (-7.6934, -26.2573) (-7.6834, -26.2308) (-7.6741, -26.204) (-7.6653, -26.177) (-7.6567, -26.1498) (-7.6483, -26.1226) (-7.64, -26.0953) (-7.632, -26.0678) (-7.6243, -26.0403) (-7.6169, -26.0126) (-7.6098, -25.9847) (-7.6031, -25.9567) (-7.5967, -25.9286) (-7.5906, -25.9003) (-7.5846, -25.872) (-7.5789, -25.8436) (-7.5733, -25.8151) (-7.5679, -25.7866) (-7.5628, -25.7579) (-7.5579, -25.7292) (-7.5532, -25.7004) (-7.5487, -25.6715) (-7.5444, -25.6425) (-7.5403, -25.6134) (-7.5364, -25.5843) (-7.5327, -25.5551) (-7.5292, -25.5258) (-7.5259, -25.4964) (-7.5227, -25.467) (-7.5197, -25.4376) (-7.5169, -25.408) (-7.5143, -25.3784) (-7.5119, -25.3487) (-7.5096, -25.319) (-7.5075, -25.2892) (-7.5056, -25.2594) (-7.5038, -25.2295) (-7.5022, -25.1996) (-7.5008, -25.1696) (-7.4996, -25.1395) (-7.4985, -25.1094) (-7.4975, -25.0792) (-7.4967, -25.049) (-7.4961, -25.0188) (-7.4957, -24.9885) (-7.4954, -24.9581) (-7.4952, -24.9277) (-7.4952, -24.8973) (-7.4954, -24.8668) (-7.4957, -24.8363) (-7.4962, -24.8057) (-7.4968, -24.7751) (-7.4975, -24.7444) (-7.4985, -24.7137) (-7.4995, -24.683) (-7.5007, -24.6522) (-7.5021, -24.6214) (-7.5036, -24.5905) (-7.5053, -24.5596) (-7.5071, -24.5287) (-7.509, -24.4977) (-7.5111, -24.4667) (-7.5133, -24.4357) (-7.5157, -24.4046) (-7.5182, -24.3736) (-7.5209, -24.3424) (-7.5236, -24.3113) (-7.526, -24.2863) (-7.5278, -24.2676) (-7.5291, -24.2551) (-7.5297, -24.2488) knots 0 0 0 0 0 0 0.01428571 0.02857143 0.04285714 0.05714286 0.07142857 0.08571429 0.1 0.11428571 0.12857143 0.14285714 0.15714286 0.17142857 0.18571429 0.2 0.21428571 0.22857143 0.24285714 0.25714286 0.27142857 0.28571429 0.3 0.31428571 0.32857143 0.34285714 0.35714286 0.37142857 0.38571429 0.4 0.41428571 0.42857143 0.44285714 0.45714286 0.47142857 0.48571429 0.5 0.51428571 0.52857143 0.54285714 0.55714286 0.57142857 0.58571429 0.6 0.61428571 0.62857143 0.64285714 0.65714286 0.67142857 0.68571429 0.7 0.71428571 0.72857143 0.74285714 0.75714286 0.77142857 0.78571429 0.8 0.81428571 0.82857143 0.84285714 0.85714286 0.87142857 0.88571429 0.9 0.91428571 0.92857143 0.94285714 0.95714286 0.97142857 0.98571429 1 1 1 1 1 1
  arc A30 (-7.5297, -24.2488) -> (-8.2732, -23.9406) centre (-13.5, -37.5997) ccw
  spline S15 degree 5 poles (-8.2732, -23.9406) (-8.2781, -23.9446) (-8.2878, -23.9525) (-8.3024, -23.9645) (-8.3217, -23.9804) (-8.3457, -24.0005) (-8.3696, -24.0206) (-8.3934, -24.0408) (-8.417, -24.0611) (-8.4406, -24.0814) (-8.464, -24.1019) (-8.4872, -24.1224) (-8.5104, -24.143) (-8.5334, -24.1636) (-8.5563, -24.1844) (-8.5791, -24.2052) (-8.6017, -24.2261) (-8.6242, -24.247) (-8.6466, -24.2681) (-8.6688, -24.2892) (-8.6909, -24.3104) (-8.7129, -24.3317) (-8.7347, -24.353) (-8.7564, -24.3745) (-8.7779, -24.396) (-8.7993, -24.4176) (-8.8206, -24.4392) (-8.8417, -24.461) (-8.8627, -24.4828) (-8.8835, -24.5047) (-8.9042, -24.5267) (-8.9247, -24.5487) (-8.9451, -24.5708) (-8.9653, -24.5931) (-8.9853, -24.6153) (-9.0053, -24.6377) (-9.025, -24.6602) (-9.0446, -24.6827) (-9.064, -24.7053) (-9.0833, -24.728) (-9.1024, -24.7508) (-9.1213, -24.7736) (-9.1401, -24.7965) (-9.1586, -24.8196) (-9.177, -24.8427) (-9.1953, -24.8658) (-9.2133, -24.8891) (-9.2312, -24.9125) (-9.2489, -24.9359) (-9.2663, -24.9594) (-9.2836, -24.983) (-9.3007, -25.0067) (-9.3176, -25.0305) (-9.3342, -25.0544) (-9.3506, -25.0783) (-9.3668, -25.1024) (-9.3829, -25.1266) (-9.3987, -25.1508) (-9.4143, -25.1751) (-9.4297, -25.1995) (-9.4447, -25.224) (-9.4595, -25.2487) (-9.4739, -25.2735) (-9.4879, -25.2985) (-9.5016, -25.3235) (-9.5151, -25.3487) (-9.5285, -25.3739) (-9.5416, -25.3991) (-9.5545, -25.4245) (-9.5669, -25.45) (-9.5786, -25.4758) (-9.5871, -25.4968) (-9.5929, -25.5127) (-9.5965, -25.5234) (-9.5983, -25.5288) knots -1 -1 -1 -1 -1 -1 -0.98571429 -0.97142857 -0.95714286 -0.94285714 -0.92857143 -0.91428571 -0.9 -0.88571429 -0.87142857 -0.85714286 -0.84285714 -0.82857143 -0.81428571 -0.8 -0.78571429 -0.77142857 -0.75714286 -0.74285714 -0.72857143 -0.71428571 -0.7 -0.68571429 -0.67142857 -0.65714286 -0.64285714 -0.62857143 -0.61428571 -0.6 -0.58571429 -0.57142857 -0.55714286 -0.54285714 -0.52857143 -0.51428571 -0.5 -0.48571429 -0.47142857 -0.45714286 -0.44285714 -0.42857143 -0.41428571 -0.4 -0.38571429 -0.37142857 -0.35714286 -0.34285714 -0.32857143 -0.31428571 -0.3 -0.28571429 -0.27142857 -0.25714286 -0.24285714 -0.22857143 -0.21428571 -0.2 -0.18571429 -0.17142857 -0.15714286 -0.14285714 -0.12857143 -0.11428571 -0.1 -0.08571429 -0.07142857 -0.05714286 -0.04285714 -0.02857143 -0.01428571 0 0 0 0 0 0
  line L15 (-9.5983, -25.5288) -> (-9.7176, -25.8979)
  arc A31 (-9.8427, -25.9625) -> (-9.7176, -25.8979) centre (-9.8127, -25.8671) ccw
  arc A32 (-9.8427, -25.9625) -> (-10.8418, -25.6945) centre (-13.5, -37.5997) ccw
  arc A33 (-10.9178, -25.5759) -> (-10.8418, -25.6945) centre (-10.82, -25.5969) ccw
  line L16 (-10.9178, -25.5759) -> (-10.8364, -25.1967)
  spline S16 degree 5 poles (-10.8364, -25.1967) (-10.8352, -25.1911) (-10.8329, -25.18) (-10.83, -25.1633) (-10.8269, -25.1409) (-10.8241, -25.1128) (-10.822, -25.0845) (-10.8205, -25.0561) (-10.8193, -25.0276) (-10.8182, -24.9991) (-10.8173, -24.9706) (-10.8166, -24.942) (-10.8163, -24.9134) (-10.8163, -24.8847) (-10.8167, -24.856) (-10.8175, -24.8272) (-10.8186, -24.7984) (-10.82, -24.7695) (-10.8215, -24.7406) (-10.8233, -24.7117) (-10.8253, -24.6827) (-10.8275, -24.6538) (-10.83, -24.6248) (-10.8326, -24.5957) (-10.8356, -24.5667) (-10.8387, -24.5376) (-10.8421, -24.5085) (-10.8457, -24.4793) (-10.8495, -24.4502) (-10.8534, -24.421) (-10.8576, -24.3918) (-10.862, -24.3626) (-10.8665, -24.3334) (-10.8713, -24.3042) (-10.8762, -24.2749) (-10.8814, -24.2456) (-10.8867, -24.2163) (-10.8922, -24.1871) (-10.8979, -24.1577) (-10.9038, -24.1284) (-10.9098, -24.0991) (-10.916, -24.0698) (-10.9224, -24.0404) (-10.929, -24.011) (-10.9357, -23.9817) (-10.9426, -23.9523) (-10.9497, -23.9229) (-10.9569, -23.8935) (-10.9643, -23.8641) (-10.9719, -23.8348) (-10.9796, -23.8054) (-10.9875, -23.7759) (-10.9955, -23.7465) (-11.0037, -23.7171) (-11.0121, -23.6877) (-11.0206, -23.6583) (-11.0293, -23.6289) (-11.0381, -23.5995) (-11.0471, -23.5701) (-11.0562, -23.5406) (-11.0655, -23.5112) (-11.075, -23.4818) (-11.0846, -23.4524) (-11.0943, -23.423) (-11.1042, -23.3936) (-11.1142, -23.3642) (-11.1244, -23.3348) (-11.1347, -23.3054) (-11.1452, -23.276) (-11.1558, -23.2466) (-11.1666, -23.2173) (-11.1753, -23.1938) (-11.1819, -23.1761) (-11.1864, -23.1644) (-11.1886, -23.1585) knots 0 0 0 0 0 0 0.01428571 0.02857143 0.04285714 0.05714286 0.07142857 0.08571429 0.1 0.11428571 0.12857143 0.14285714 0.15714286 0.17142857 0.18571429 0.2 0.21428571 0.22857143 0.24285714 0.25714286 0.27142857 0.28571429 0.3 0.31428571 0.32857143 0.34285714 0.35714286 0.37142857 0.38571429 0.4 0.41428571 0.42857143 0.44285714 0.45714286 0.47142857 0.48571429 0.5 0.51428571 0.52857143 0.54285714 0.55714286 0.57142857 0.58571429 0.6 0.61428571 0.62857143 0.64285714 0.65714286 0.67142857 0.68571429 0.7 0.71428571 0.72857143 0.74285714 0.75714286 0.77142857 0.78571429 0.8 0.81428571 0.82857143 0.84285714 0.85714286 0.87142857 0.88571429 0.9 0.91428571 0.92857143 0.94285714 0.95714286 0.97142857 0.98571429 1 1 1 1 1 1
  arc A34 (-11.1886, -23.1585) -> (-11.9866, -23.0532) centre (-13.5, -37.5997) ccw
  spline S17 degree 5 poles (-11.9866, -23.0532) (-11.9902, -23.0583) (-11.9976, -23.0685) (-12.0085, -23.0838) (-12.023, -23.1043) (-12.0411, -23.1298) (-12.0589, -23.1555) (-12.0767, -23.1811) (-12.0943, -23.2068) (-12.1117, -23.2326) (-12.1291, -23.2584) (-12.1462, -23.2842) (-12.1633, -23.3101) (-12.1802, -23.336) (-12.1969, -23.3619) (-12.2135, -23.3879) (-12.23, -23.414) (-12.2463, -23.4401) (-12.2624, -23.4662) (-12.2784, -23.4923) (-12.2943, -23.5185) (-12.31, -23.5448) (-12.3256, -23.571) (-12.341, -23.5974) (-12.3562, -23.6237) (-12.3713, -23.6501) (-12.3862, -23.6765) (-12.401, -23.703) (-12.4156, -23.7295) (-12.43, -23.756) (-12.4443, -23.7826) (-12.4584, -23.8092) (-12.4724, -23.8359) (-12.4862, -23.8626) (-12.4998, -23.8893) (-12.5132, -23.9161) (-12.5265, -23.9429) (-12.5396, -23.9697) (-12.5525, -23.9966) (-12.5652, -24.0235) (-12.5778, -24.0504) (-12.5902, -24.0774) (-12.6023, -24.1044) (-12.6143, -24.1314) (-12.6261, -24.1585) (-12.6377, -24.1856) (-12.6491, -24.2127) (-12.6603, -24.2399) (-12.6713, -24.2671) (-12.6822, -24.2944) (-12.6927, -24.3216) (-12.7031, -24.3489) (-12.7132, -24.3763) (-12.7231, -24.4037) (-12.7328, -24.4311) (-12.7422, -24.4585) (-12.7514, -24.486) (-12.7604, -24.5135) (-12.7692, -24.541) (-12.7778, -24.5686) (-12.786, -24.5962) (-12.7938, -24.6238) (-12.8013, -24.6515) (-12.8084, -24.6792) (-12.8152, -24.707) (-12.8217, -24.7348) (-12.8281, -24.7626) (-12.8342, -24.7904) (-12.8401, -24.8182) (-12.8455, -24.8461) (-12.8501, -24.874) (-12.8529, -24.8964) (-12.8544, -24.9133) (-12.8551, -24.9246) (-12.8554, -24.9303) knots -1 -1 -1 -1 -1 -1 -0.98571429 -0.97142857 -0.95714286 -0.94285714 -0.92857143 -0.91428571 -0.9 -0.88571429 -0.87142857 -0.85714286 -0.84285714 -0.82857143 -0.81428571 -0.8 -0.78571429 -0.77142857 -0.75714286 -0.74285714 -0.72857143 -0.71428571 -0.7 -0.68571429 -0.67142857 -0.65714286 -0.64285714 -0.62857143 -0.61428571 -0.6 -0.58571429 -0.57142857 -0.55714286 -0.54285714 -0.52857143 -0.51428571 -0.5 -0.48571429 -0.47142857 -0.45714286 -0.44285714 -0.42857143 -0.41428571 -0.4 -0.38571429 -0.37142857 -0.35714286 -0.34285714 -0.32857143 -0.31428571 -0.3 -0.28571429 -0.27142857 -0.25714286 -0.24285714 -0.22857143 -0.21428571 -0.2 -0.18571429 -0.17142857 -0.15714286 -0.14285714 -0.12857143 -0.11428571 -0.1 -0.08571429 -0.07142857 -0.05714286 -0.04285714 -0.02857143 -0.01428571 0 0 0 0 0 0
  line L17 (-12.8554, -24.9303) -> (-12.8751, -25.3176)
  arc A35 (-12.9792, -25.4125) -> (-12.8751, -25.3176) centre (-12.975, -25.3126) ccw
  arc A36 (-12.9792, -25.4125) -> (-14.0137, -25.4122) centre (-13.5, -37.5997) ccw
  arc A37 (-14.1178, -25.3173) -> (-14.0137, -25.4122) centre (-14.0179, -25.3123) ccw
  line L18 (-14.1178, -25.3173) -> (-14.1373, -24.9299)
  spline S18 degree 5 poles (-14.1373, -24.9299) (-14.1376, -24.9242) (-14.1383, -24.9129) (-14.1397, -24.8961) (-14.1425, -24.8736) (-14.1471, -24.8457) (-14.1525, -24.8178) (-14.1584, -24.79) (-14.1645, -24.7622) (-14.1708, -24.7344) (-14.1773, -24.7066) (-14.1841, -24.6788) (-14.1912, -24.6511) (-14.1986, -24.6234) (-14.2065, -24.5957) (-14.2147, -24.5681) (-14.2232, -24.5406) (-14.232, -24.513) (-14.241, -24.4855) (-14.2502, -24.4581) (-14.2596, -24.4306) (-14.2692, -24.4032) (-14.2791, -24.3758) (-14.2892, -24.3485) (-14.2996, -24.3212) (-14.3101, -24.2939) (-14.3209, -24.2666) (-14.3319, -24.2394) (-14.3431, -24.2122) (-14.3545, -24.1851) (-14.3661, -24.158) (-14.3779, -24.1309) (-14.3898, -24.1038) (-14.402, -24.0768) (-14.4144, -24.0499) (-14.4269, -24.0229) (-14.4396, -23.996) (-14.4525, -23.9691) (-14.4656, -23.9423) (-14.4789, -23.9155) (-14.4923, -23.8887) (-14.5059, -23.862) (-14.5196, -23.8353) (-14.5336, -23.8086) (-14.5477, -23.782) (-14.5619, -23.7554) (-14.5764, -23.7289) (-14.591, -23.7024) (-14.6057, -23.6759) (-14.6206, -23.6495) (-14.6357, -23.6231) (-14.6509, -23.5967) (-14.6663, -23.5704) (-14.6819, -23.5441) (-14.6975, -23.5178) (-14.7134, -23.4916) (-14.7294, -23.4655) (-14.7455, -23.4393) (-14.7618, -23.4132) (-14.7783, -23.3872) (-14.7948, -23.3612) (-14.8116, -23.3352) (-14.8284, -23.3093) (-14.8455, -23.2834) (-14.8626, -23.2576) (-14.8799, -23.2318) (-14.8974, -23.206) (-14.915, -23.1803) (-14.9327, -23.1546) (-14.9506, -23.129) (-14.9686, -23.1034) (-14.9831, -23.083) (-14.994, -23.0677) (-15.0013, -23.0575) (-15.005, -23.0524) knots 0 0 0 0 0 0 0.01428571 0.02857143 0.04285714 0.05714286 0.07142857 0.08571429 0.1 0.11428571 0.12857143 0.14285714 0.15714286 0.17142857 0.18571429 0.2 0.21428571 0.22857143 0.24285714 0.25714286 0.27142857 0.28571429 0.3 0.31428571 0.32857143 0.34285714 0.35714286 0.37142857 0.38571429 0.4 0.41428571 0.42857143 0.44285714 0.45714286 0.47142857 0.48571429 0.5 0.51428571 0.52857143 0.54285714 0.55714286 0.57142857 0.58571429 0.6 0.61428571 0.62857143 0.64285714 0.65714286 0.67142857 0.68571429 0.7 0.71428571 0.72857143 0.74285714 0.75714286 0.77142857 0.78571429 0.8 0.81428571 0.82857143 0.84285714 0.85714286 0.87142857 0.88571429 0.9 0.91428571 0.92857143 0.94285714 0.95714286 0.97142857 0.98571429 1 1 1 1 1 1
  arc A38 (-15.005, -23.0524) -> (-15.803, -23.1572) centre (-13.5, -37.5997) ccw